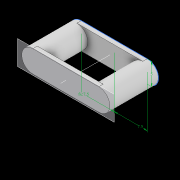
# Autodesk Inventor part: Part1
Saved by Autodesk Inventor 2022.2 (Build 262287010, 287A)
## iProperties
Created: 2022-05-28
Part Number: Part1
Material: Generic
Document SubType Name: Modeling
Designer: Árni Þór Þorgeirsson
Density: 1 g/cm^3
Appearance: Default
Author: Árni Þór Þorgeirsson
Autodesk Inventor part; units mm, degrees
ref_plane "YZ Plane" through (0, 0, 0) normal (1, 0, 0) x (0, 1, 0)
ref_plane "XZ Plane" through (0, 0, 0) normal (0, 1, 0) x (-1, 0, 0)
sketch "Sketch1" plane through (0, 0, 0) normal (0, 0, 1) x (1, 0, 0)
  line L0 (-7.5, 2.5) -> (7.5, 2.5)
  line L1 (7.5, -2.5) -> (-7.5, -2.5)
  line L2 (-7.5, 2.5) -> (7.5, -2.5) construction
  line L3 (7.5, 2.5) -> (-7.5, -2.5) construction
  circle A0 centre (-7.5, 0) radius 2.5
  circle A1 centre (7.5, 0) radius 2.5
  point P0 (0, 0)
  point P1 (0, 0)
  point P2 (0, 0)
  dimension "d1" = 5
  dimension "d9" = 7.5
  dimension "d10" = 7.5
  constraints: 8 end point, 4 midpoint, 4 point on circle, 4 tangent, 2 centre point, 1 horizontal, 1 parallel
  measures "d1" distance of L3.start L2.end
  measures "d9" distance of A0.centre point (0, 0)
  measures "d10" distance of A1.centre point (0, 0)
extrude "Extrusion1" add sketch "Sketch1" along normal blind 1
extrude "Extrusion2" add sketch "Sketch1" along normal blind 10 contours A0 | A1
ref_plane "Work Plane1" through (0, 0, 11) normal (0, 0, 1) x (1, 0, 0)
sketch "Sketch2" plane through (0, 0, 11) normal (0, 0, 1) x (1, 0, 0)
  arc A0 (7.5, 2.5) -> (7.5, -2.5) centre (7.5, 0) ccw projected
  line L0 (7.5, 2.5) -> (-7.5, 2.5) projected
  arc A1 (-7.5, -2.5) -> (-7.5, 2.5) centre (-7.5, 0) ccw projected
  line L1 (-7.5, -2.5) -> (7.5, -2.5) projected
  circle A2 centre (-7.5, 0) radius 2.5 projected
  circle A3 centre (7.5, 0) radius 2.5 projected
  point P0 (0, 0)
  point P1 (-7.5, -2.5)
  point P2 (7.5, -2.5)
extrude "Extrusion3" add sketch "Sketch2" against normal blind 1
equation "\"d9\" = d10"
body "Solid1"
